bed levelling_v5 (Autodesk Fusion 360 design; units mm, degrees)
Autodesk Fusion 360 part; units mm, degrees
sketch "Sketch1" plane through (0, 0, 0) normal (0, 0, 1) x (1, 0, 0)
  line L0 (-27, 15.5) -> (27, 15.5)
  line L1 (27, 15.5) -> (27, -15.5)
  line L2 (27, -15.5) -> (-27, -15.5)
  line L3 (-27, -15.5) -> (-27, 15.5)
  line L4 (-27, 15.5) -> (27, -15.5) construction
  line L5 (27, 15.5) -> (-27, -15.5) construction
  dimension "d1" = 31
  dimension "d2" = 54
  constraint horizontal L0
  constraint perpendicular L0 L1
  constraint parallel L0 L2
  constraint parallel L1 L3
  constraint coincident L4 origin
  constraint coincident L5 origin
  measures "d1" distance of L0.start L2.end
  measures "d2" distance of L0.start L0.end
extrude "Extrude1" add sketch "Sketch1" along normal blind 0.5
